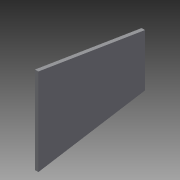
# Autodesk Inventor part: Part17
Saved by Autodesk Inventor 2015 (Build 190159000, 159)
## iProperties
Created: 2014-10-18
Part Number: Part17
Material: Generic
Document SubType Name: Modeling
Designer: jesse
Density: 1 g/cm^3
Appearance: Default
Author: jesse
Autodesk Inventor part; units mm, degrees
ref_plane "YZ Plane" through (0, 0, 0) normal (1, 0, 0) x (0, 1, 0)
ref_plane "XZ Plane" through (0, 0, 0) normal (0, 1, 0) x (-1, 0, 0)
ref_plane "XY Plane" through (0, 0, 0) normal (0, 0, 1) x (1, 0, 0)
sketch "Sketch3" plane through (0, 0, 0) normal (1, 0, 0) x (0, 1, 0)
  line L0 (0, 155.5521) -> (-254, 155.5521)
  line L1 (-254, 155.5521) -> (-254, 0)
  line L2 (-254, 0) -> (0, 0)
  line L3 (0, 0) -> (0, 155.5521)
  dimension "d0" = 254
  constraints: 8 end point, 2 parallel, 1 horizontal, 1 perpendicular
  measures "d0" distance of L2.end L1.end
extrude "Extrusion1" add sketch "Sketch3" along normal blind 5
sketch "Sketch4" plane through (0, 0, 0) normal (-1, 0, 0) x (0, 0, 1)
  line L0 (155.5521, 0) -> (155.5521, -254) construction
  line L1 (0, 0) -> (155.5521, 0) projected
  line L2 (0, -254) -> (0, 0) construction
  line L3 (155.5521, -254) -> (0, -254) projected
  line L4 (0, 0) -> (0, -88.9)
  line L5 (0, -254) -> (0, 0) projected
  line L6 (155.5521, 0) -> (0, 0)
  line L7 (155.5521, -254) -> (0, -254)
  line L8 (0, -254) -> (0, -165.1)
  line L9 (155.5521, -254) -> (155.5521, -190.5)
  line L10 (155.5521, 0) -> (155.5521, -254) projected
  line L11 (155.5521, -190.5) -> (0, -165.1)
  line L12 (155.5521, 0) -> (155.5521, -63.5)
  line L13 (155.5521, -63.5) -> (0, -88.9)
  dimension "d3" = 88.9
  dimension "d4" = 88.9
  dimension "d5" = 63.5
  dimension "d7" = 63.5
  dimension "d10" = 155.5521
  constraints: 16 end point, 4 point on line, 2 perpendicular
  measures "d3" distance of L1.start L4.end
  measures "d4" distance of L2.start L8.end
  measures "d5" distance of L0.end L9.end
  measures "d7" distance of L0.start L12.end
  measures "d10" horizontal distance of L4.end L12.end
extrude "Extrusion2" cut sketch "Sketch4" against normal through all contours L1 L10 L13 L4 | L11 L9 L3 L5
sketch "Sketch7" plane through (5, 0, 0) normal (1, 0, 0) x (0, 0, -1)
  line L0 (-155.5521, -190.5) -> (0, -165.1) projected
  line L1 (0, -165.1) -> (0, -88.9) projected
  line L2 (0, -88.9) -> (-155.5521, -63.5) projected
  line L3 (-155.5521, -63.5) -> (-155.5521, -190.5) projected
  line L4 (0, -88.9) -> (-155.5521, -63.5)
  line L5 (-155.5521, -63.5) -> (-155.5521, -68.5)
  line L6 (-155.5521, -63.5) -> (-155.5521, -190.5) projected
  line L7 (0, -88.9) -> (0, -93.9)
  line L8 (0, -165.1) -> (0, -88.9) projected
  line L9 (0, -93.9) -> (-155.5521, -68.5)
  line L10 (-155.5521, -190.5) -> (-155.5521, -185.5)
  line L11 (-155.5521, -185.5) -> (0, -160.1)
  line L12 (0, -165.1) -> (-154.7568, -190.3701)
  line L13 (0, -165.1) -> (-155.5521, -190.5) projected
  point P0 (0, 0)
  dimension "d14" = 5
  dimension "d15" = 5
  constraints: 14 end point, 5 point on line, 2 parallel
  measures "d14" distance of L1.end L7.end
  measures "d15" distance of L0.start L10.end
extrude "Extrusion3" add sketch "Sketch7" along normal blind 38.1 contours L3 L11 L1 L0 | L3 L2 L1 L9
body "Solid1"
